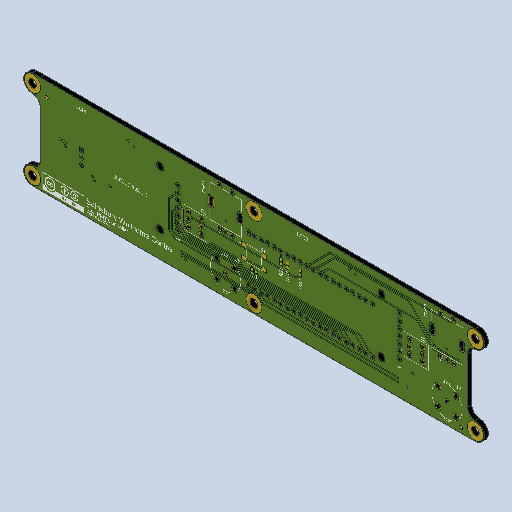
# Autodesk Inventor part: Dual PMT Controller_BOARD
Saved by Autodesk Inventor 2023 (Build 270158000, 158)
## iProperties
Created: 2023-07-11
Part Number: Dual PMT Controller_BOARD
Material: Generic
Document SubType Name: Modeling
Designer: Graeme
Density: 1 g/cm^3
Appearance: BoardColor
Author: Graeme
Autodesk Inventor part; units mm, degrees
ref_plane "YZ Plane" through (0, 0, 0) normal (1, 0, 0) x (0, 1, 0)
ref_plane "XZ Plane" through (0, 0, 0) normal (0, 1, 0) x (-1, 0, 0)
ref_plane "BoardFrontPlane" through (0, 0, 0) normal (0, 0, 1) x (1, 0, 0)
sketch "Sketch1" plane through (0, 0, 0) normal (0, 0, 1) x (1, 0, 0)
  line L0 (25, 25) -> (28, 25)
  line L1 (28, 25) -> (194, 25)
  line L2 (194, 25) -> (197, 25)
  arc A0 (197, 25) -> (197, 32) centre (197, 28.5) ccw
  arc A1 (194, 35) -> (197, 32) centre (197, 35) ccw
  line L3 (194, 35) -> (194, 53)
  arc A2 (197, 56) -> (194, 53) centre (197, 53) ccw
  arc A3 (197, 56) -> (197, 63) centre (197, 59.5) ccw
  line L4 (197, 63) -> (194, 63)
  line L5 (194, 63) -> (28, 63)
  line L6 (28, 63) -> (25, 63)
  arc A4 (25, 63) -> (25, 56) centre (25, 59.5) ccw
  arc A5 (28, 53) -> (25, 56) centre (25, 53) ccw
  line L7 (28, 53) -> (28, 35)
  arc A6 (25, 32) -> (28, 35) centre (25, 35) ccw
  arc A7 (25, 32) -> (25, 25) centre (25, 28.5) ccw
  constraints: 16 end point, 16 point on circle, 8 centre point
extrude "BoardOutline" add sketch "Sketch1" along normal blind 1.5954
sketch "Sketch4" plane through (0, 0, 1.5954) normal (0, 0, 1) x (1, 0, 0)
  line L0 (105.7, 53.45) -> (105.7, 55.55) construction
  line L1 (106.4, 53.45) -> (106.4, 55.55)
  line L2 (105, 55.55) -> (105, 53.45)
  arc A0 (105, 53.45) -> (106.4, 53.45) centre (105.7, 53.45) ccw
  arc A1 (106.4, 55.55) -> (105, 55.55) centre (105.7, 55.55) ccw
  point P0 (105.7, 54.5)
  constraints: 8 end point, 4 point on circle, 4 tangent, 2 centre point, 1 midpoint, 1 parallel
extrude "ENC1-4" cut sketch "Sketch4" against normal through all
sketch "Sketch5" plane through (0, 0, 1.5954) normal (0, 0, 1) x (1, 0, 0)
  line L0 (94.3, 53.45) -> (94.3, 55.55) construction
  line L1 (95, 53.45) -> (95, 55.55)
  line L2 (93.6, 55.55) -> (93.6, 53.45)
  arc A0 (93.6, 53.45) -> (95, 53.45) centre (94.3, 53.45) ccw
  arc A1 (95, 55.55) -> (93.6, 55.55) centre (94.3, 55.55) ccw
  point P0 (94.3, 54.5)
  constraints: 8 end point, 4 point on circle, 4 tangent, 2 centre point, 1 midpoint, 1 parallel
extrude "ENC1-3" cut sketch "Sketch5" against normal through all
sketch "Sketch6" plane through (0, 0, 1.5954) normal (0, 0, 1) x (1, 0, 0)
  point P0 (102.5, 47)
hole "ENC1-B" at (102.5, 47, 1.5954) direction (0, 0, -1) diameter 1 end through all
sketch "Sketch7" plane through (0, 0, 1.5954) normal (0, 0, 1) x (1, 0, 0)
  point P0 (100, 47)
hole "ENC1-C" at (100, 47, 1.5954) direction (0, 0, -1) diameter 1 end through all
sketch "Sketch8" plane through (0, 0, 1.5954) normal (0, 0, 1) x (1, 0, 0)
  point P0 (97.5, 47)
hole "ENC1-A" at (97.5, 47, 1.5954) direction (0, 0, -1) diameter 1 end through all
sketch "Sketch9" plane through (0, 0, 1.5954) normal (0, 0, 1) x (1, 0, 0)
  point P0 (102.5, 61.5)
hole "ENC1-2" at (102.5, 61.5, 1.5954) direction (0, 0, -1) diameter 1 end through all
sketch "Sketch10" plane through (0, 0, 1.5954) normal (0, 0, 1) x (1, 0, 0)
  point P0 (97.5, 61.5)
hole "ENC1-1" at (97.5, 61.5, 1.5954) direction (0, 0, -1) diameter 1 end through all
sketch "Sketch11" plane through (0, 0, 1.5954) normal (0, 0, 1) x (1, 0, 0)
  line L0 (191.7, 53.45) -> (191.7, 55.55) construction
  line L1 (192.4, 53.45) -> (192.4, 55.55)
  line L2 (191, 55.55) -> (191, 53.45)
  arc A0 (191, 53.45) -> (192.4, 53.45) centre (191.7, 53.45) ccw
  arc A1 (192.4, 55.55) -> (191, 55.55) centre (191.7, 55.55) ccw
  point P0 (191.7, 54.5)
  constraints: 8 end point, 4 point on circle, 4 tangent, 2 centre point, 1 midpoint, 1 parallel
extrude "ENC2-4" cut sketch "Sketch11" against normal through all
sketch "Sketch12" plane through (0, 0, 1.5954) normal (0, 0, 1) x (1, 0, 0)
  line L0 (180.3, 53.45) -> (180.3, 55.55) construction
  line L1 (181, 53.45) -> (181, 55.55)
  line L2 (179.6, 55.55) -> (179.6, 53.45)
  arc A0 (179.6, 53.45) -> (181, 53.45) centre (180.3, 53.45) ccw
  arc A1 (181, 55.55) -> (179.6, 55.55) centre (180.3, 55.55) ccw
  point P0 (180.3, 54.5)
  constraints: 8 end point, 4 point on circle, 4 tangent, 2 centre point, 1 midpoint, 1 parallel
extrude "ENC2-3" cut sketch "Sketch12" against normal through all
sketch "Sketch13" plane through (0, 0, 1.5954) normal (0, 0, 1) x (1, 0, 0)
  point P0 (188.5, 47)
hole "ENC2-B" at (188.5, 47, 1.5954) direction (0, 0, -1) diameter 1 end through all
sketch "Sketch14" plane through (0, 0, 1.5954) normal (0, 0, 1) x (1, 0, 0)
  point P0 (186, 47)
hole "ENC2-C" at (186, 47, 1.5954) direction (0, 0, -1) diameter 1 end through all
sketch "Sketch15" plane through (0, 0, 1.5954) normal (0, 0, 1) x (1, 0, 0)
  point P0 (183.5, 47)
hole "ENC2-A" at (183.5, 47, 1.5954) direction (0, 0, -1) diameter 1 end through all
sketch "Sketch16" plane through (0, 0, 1.5954) normal (0, 0, 1) x (1, 0, 0)
  point P0 (188.5, 61.5)
hole "ENC2-2" at (188.5, 61.5, 1.5954) direction (0, 0, -1) diameter 1 end through all
sketch "Sketch17" plane through (0, 0, 1.5954) normal (0, 0, 1) x (1, 0, 0)
  point P0 (183.5, 61.5)
hole "ENC2-1" at (183.5, 61.5, 1.5954) direction (0, 0, -1) diameter 1 end through all
sketch "Sketch18" plane through (0, 0, 1.5954) normal (0, 0, 1) x (1, 0, 0)
  point P0 (100, 33)
hole "J9-1" at (100, 33, 1.5954) direction (0, 0, -1) diameter 0.9906 end through all
sketch "Sketch19" plane through (0, 0, 1.5954) normal (0, 0, 1) x (1, 0, 0)
  point P0 (96.5583, 36.4417)
hole "J9-2" at (96.5583, 36.4417, 1.5954) direction (0, 0, -1) diameter 1.4986 end through all
sketch "Sketch20" plane through (0, 0, 1.5954) normal (0, 0, 1) x (1, 0, 0)
  point P0 (103.4417, 36.4417)
hole "J9-3" at (103.4417, 36.4417, 1.5954) direction (0, 0, -1) diameter 1.4986 end through all
sketch "Sketch21" plane through (0, 0, 1.5954) normal (0, 0, 1) x (1, 0, 0)
  point P0 (96.5583, 29.5583)
hole "J9-4" at (96.5583, 29.5583, 1.5954) direction (0, 0, -1) diameter 1.4986 end through all
sketch "Sketch22" plane through (0, 0, 1.5954) normal (0, 0, 1) x (1, 0, 0)
  point P0 (103.4417, 29.5583)
hole "J9-5" at (103.4417, 29.5583, 1.5954) direction (0, 0, -1) diameter 1.4986 end through all
sketch "Sketch23" plane through (0, 0, 1.5954) normal (0, 0, 1) x (1, 0, 0)
  point P0 (186, 33)
hole "J7-1" at (186, 33, 1.5954) direction (0, 0, -1) diameter 0.9906 end through all
sketch "Sketch24" plane through (0, 0, 1.5954) normal (0, 0, 1) x (1, 0, 0)
  point P0 (182.5583, 36.4417)
hole "J7-2" at (182.5583, 36.4417, 1.5954) direction (0, 0, -1) diameter 1.4986 end through all
sketch "Sketch25" plane through (0, 0, 1.5954) normal (0, 0, 1) x (1, 0, 0)
  point P0 (189.4417, 36.4417)
hole "J7-3" at (189.4417, 36.4417, 1.5954) direction (0, 0, -1) diameter 1.4986 end through all
sketch "Sketch26" plane through (0, 0, 1.5954) normal (0, 0, 1) x (1, 0, 0)
  point P0 (182.5583, 29.5583)
hole "J7-4" at (182.5583, 29.5583, 1.5954) direction (0, 0, -1) diameter 1.4986 end through all
sketch "Sketch27" plane through (0, 0, 1.5954) normal (0, 0, 1) x (1, 0, 0)
  point P0 (189.4417, 29.5583)
hole "J7-5" at (189.4417, 29.5583, 1.5954) direction (0, 0, -1) diameter 1.4986 end through all
sketch "Sketch28" plane through (0, 0, 1.5954) normal (0, 0, 1) x (1, 0, 0)
  point P0 (85.5, 41.46)
hole "S3-1" at (85.5, 41.46, 1.5954) direction (0, 0, -1) diameter 1.09 end through all
sketch "Sketch29" plane through (0, 0, 1.5954) normal (0, 0, 1) x (1, 0, 0)
  point P0 (85.5, 44)
hole "S3-2" at (85.5, 44, 1.5954) direction (0, 0, -1) diameter 1.09 end through all
sketch "Sketch30" plane through (0, 0, 1.5954) normal (0, 0, 1) x (1, 0, 0)
  point P0 (85.5, 46.54)
hole "S3-3" at (85.5, 46.54, 1.5954) direction (0, 0, -1) diameter 1.09 end through all
sketch "Sketch31" plane through (0, 0, 1.5954) normal (0, 0, 1) x (1, 0, 0)
  point P0 (90.58, 41.46)
hole "S3-4" at (90.58, 41.46, 1.5954) direction (0, 0, -1) diameter 1.09 end through all
sketch "Sketch32" plane through (0, 0, 1.5954) normal (0, 0, 1) x (1, 0, 0)
  point P0 (90.58, 44)
hole "S3-5" at (90.58, 44, 1.5954) direction (0, 0, -1) diameter 1.09 end through all
sketch "Sketch33" plane through (0, 0, 1.5954) normal (0, 0, 1) x (1, 0, 0)
  point P0 (90.58, 46.54)
hole "S3-6" at (90.58, 46.54, 1.5954) direction (0, 0, -1) diameter 1.09 end through all
sketch "Sketch34" plane through (0, 0, 1.5954) normal (0, 0, 1) x (1, 0, 0)
  point P0 (171.5, 41.46)
hole "S2-1" at (171.5, 41.46, 1.5954) direction (0, 0, -1) diameter 1.09 end through all
sketch "Sketch35" plane through (0, 0, 1.5954) normal (0, 0, 1) x (1, 0, 0)
  point P0 (171.5, 44)
hole "S2-2" at (171.5, 44, 1.5954) direction (0, 0, -1) diameter 1.09 end through all
sketch "Sketch36" plane through (0, 0, 1.5954) normal (0, 0, 1) x (1, 0, 0)
  point P0 (171.5, 46.54)
hole "S2-3" at (171.5, 46.54, 1.5954) direction (0, 0, -1) diameter 1.09 end through all
sketch "Sketch37" plane through (0, 0, 1.5954) normal (0, 0, 1) x (1, 0, 0)
  point P0 (176.58, 41.46)
hole "S2-4" at (176.58, 41.46, 1.5954) direction (0, 0, -1) diameter 1.09 end through all
sketch "Sketch38" plane through (0, 0, 1.5954) normal (0, 0, 1) x (1, 0, 0)
  point P0 (176.58, 44)
hole "S2-5" at (176.58, 44, 1.5954) direction (0, 0, -1) diameter 1.09 end through all
sketch "Sketch39" plane through (0, 0, 1.5954) normal (0, 0, 1) x (1, 0, 0)
  point P0 (176.58, 46.54)
hole "S2-6" at (176.58, 46.54, 1.5954) direction (0, 0, -1) diameter 1.09 end through all
sketch "Sketch40" plane through (0, 0, 1.5954) normal (0, 0, 1) x (1, 0, 0)
  point P0 (81.48, 53.38)
hole "LCD1-7" at (81.48, 53.38, 1.5954) direction (0, 0, -1) diameter 1 end through all
sketch "Sketch41" plane through (0, 0, 1.5954) normal (0, 0, 1) x (1, 0, 0)
  point P0 (81.48, 50.84)
hole "LCD1-6" at (81.48, 50.84, 1.5954) direction (0, 0, -1) diameter 1 end through all
sketch "Sketch42" plane through (0, 0, 1.5954) normal (0, 0, 1) x (1, 0, 0)
  point P0 (81.48, 48.3)
hole "LCD1-5" at (81.48, 48.3, 1.5954) direction (0, 0, -1) diameter 1 end through all
sketch "Sketch43" plane through (0, 0, 1.5954) normal (0, 0, 1) x (1, 0, 0)
  point P0 (81.48, 45.76)
hole "LCD1-4" at (81.48, 45.76, 1.5954) direction (0, 0, -1) diameter 1 end through all
sketch "Sketch44" plane through (0, 0, 1.5954) normal (0, 0, 1) x (1, 0, 0)
  point P0 (81.48, 43.22)
hole "LCD1-3" at (81.48, 43.22, 1.5954) direction (0, 0, -1) diameter 1 end through all
sketch "Sketch45" plane through (0, 0, 1.5954) normal (0, 0, 1) x (1, 0, 0)
  point P0 (81.48, 40.68)
hole "LCD1-2" at (81.48, 40.68, 1.5954) direction (0, 0, -1) diameter 1 end through all
sketch "Sketch46" plane through (0, 0, 1.5954) normal (0, 0, 1) x (1, 0, 0)
  point P0 (81.48, 38.14)
hole "LCD1-1" at (81.48, 38.14, 1.5954) direction (0, 0, -1) diameter 1 end through all
sketch "Sketch47" plane through (0, 0, 1.5954) normal (0, 0, 1) x (1, 0, 0)
  point P0 (74.58, 56.36)
hole "LCD1-MH1" at (74.58, 56.36, 1.5954) direction (0, 0, -1) diameter 2.5 end through all
sketch "Sketch48" plane through (0, 0, 1.5954) normal (0, 0, 1) x (1, 0, 0)
  point P0 (74.58, 35.16)
hole "LCD1-MH2" at (74.58, 35.16, 1.5954) direction (0, 0, -1) diameter 2.5 end through all
sketch "Sketch49" plane through (0, 0, 1.5954) normal (0, 0, 1) x (1, 0, 0)
  point P0 (167.48, 53.38)
hole "LCD2-7" at (167.48, 53.38, 1.5954) direction (0, 0, -1) diameter 1 end through all
sketch "Sketch50" plane through (0, 0, 1.5954) normal (0, 0, 1) x (1, 0, 0)
  point P0 (167.48, 50.84)
hole "LCD2-6" at (167.48, 50.84, 1.5954) direction (0, 0, -1) diameter 1 end through all
sketch "Sketch51" plane through (0, 0, 1.5954) normal (0, 0, 1) x (1, 0, 0)
  point P0 (167.48, 48.3)
hole "LCD2-5" at (167.48, 48.3, 1.5954) direction (0, 0, -1) diameter 1 end through all
sketch "Sketch52" plane through (0, 0, 1.5954) normal (0, 0, 1) x (1, 0, 0)
  point P0 (167.48, 45.76)
hole "LCD2-4" at (167.48, 45.76, 1.5954) direction (0, 0, -1) diameter 1 end through all
sketch "Sketch53" plane through (0, 0, 1.5954) normal (0, 0, 1) x (1, 0, 0)
  point P0 (167.48, 43.22)
hole "LCD2-3" at (167.48, 43.22, 1.5954) direction (0, 0, -1) diameter 1 end through all
sketch "Sketch54" plane through (0, 0, 1.5954) normal (0, 0, 1) x (1, 0, 0)
  point P0 (167.48, 40.68)
hole "LCD2-2" at (167.48, 40.68, 1.5954) direction (0, 0, -1) diameter 1 end through all
sketch "Sketch55" plane through (0, 0, 1.5954) normal (0, 0, 1) x (1, 0, 0)
  point P0 (167.48, 38.14)
hole "LCD2-1" at (167.48, 38.14, 1.5954) direction (0, 0, -1) diameter 1 end through all
sketch "Sketch56" plane through (0, 0, 1.5954) normal (0, 0, 1) x (1, 0, 0)
  point P0 (160.58, 56.36)
hole "LCD2-MH1" at (160.58, 56.36, 1.5954) direction (0, 0, -1) diameter 2.5 end through all
sketch "Sketch57" plane through (0, 0, 1.5954) normal (0, 0, 1) x (1, 0, 0)
  point P0 (160.58, 35.16)
hole "LCD2-MH2" at (160.58, 35.16, 1.5954) direction (0, 0, -1) diameter 2.5 end through all
sketch "Sketch98" plane through (0, 0, 1.5954) normal (0, 0, 1) x (1, 0, 0)
  point P0 (44, 46.54)
hole "PS1-1" at (44, 46.54, 1.5954) direction (0, 0, -1) diameter 0.85 end through all
sketch "Sketch99" plane through (0, 0, 1.5954) normal (0, 0, 1) x (1, 0, 0)
  point P0 (44, 44)
hole "PS1-2" at (44, 44, 1.5954) direction (0, 0, -1) diameter 0.85 end through all
sketch "Sketch100" plane through (0, 0, 1.5954) normal (0, 0, 1) x (1, 0, 0)
  point P0 (44, 41.46)
hole "PS1-3" at (44, 41.46, 1.5954) direction (0, 0, -1) diameter 0.85 end through all
sketch "Sketch101" plane through (0, 0, 1.5954) normal (0, 0, 1) x (1, 0, 0)
  point P0 (25, 59.5)
hole "Free-MH1_LWOVBYDG" at (25, 59.5, 1.5954) direction (0, 0, -1) diameter 3.1 end through all
sketch "Sketch102" plane through (0, 0, 1.5954) normal (0, 0, 1) x (1, 0, 0)
  point P0 (25, 28.5)
hole "Free-MH1_XUCMYAUQ" at (25, 28.5, 1.5954) direction (0, 0, -1) diameter 3.1 end through all
sketch "Sketch103" plane through (0, 0, 1.5954) normal (0, 0, 1) x (1, 0, 0)
  point P0 (111, 28.5)
hole "Free-MH1_AHOANEHU" at (111, 28.5, 1.5954) direction (0, 0, -1) diameter 3.1 end through all
sketch "Sketch104" plane through (0, 0, 1.5954) normal (0, 0, 1) x (1, 0, 0)
  point P0 (111, 59.5)
hole "Free-MH1_SKXHPFAL" at (111, 59.5, 1.5954) direction (0, 0, -1) diameter 3.1 end through all
sketch "Sketch105" plane through (0, 0, 1.5954) normal (0, 0, 1) x (1, 0, 0)
  point P0 (197, 28.5)
hole "Free-MH1_TQVXVKIN" at (197, 28.5, 1.5954) direction (0, 0, -1) diameter 3.1 end through all
sketch "Sketch106" plane through (0, 0, 1.5954) normal (0, 0, 1) x (1, 0, 0)
  point P0 (197, 59.5)
hole "Free-MH1_OJOGQPHQ" at (197, 59.5, 1.5954) direction (0, 0, -1) diameter 3.1 end through all
sketch "img_Top" plane through (0, 0, 1.5954) normal (0, 0, 1) x (1, 0, 0)
  line L0 (21.5, 63) -> (200.5015, 63) construction
  line L1 (200.5015, 63) -> (200.5015, 25) construction
  line L2 (200.5015, 25) -> (21.5, 25) construction
  line L3 (21.5, 25) -> (21.5, 63) construction
  constraints: 2 other
decal "Decal_Top"
sketch "img_Bottom" plane through (0, 0, -1.5954) normal (0, 0, -1) x (1, 0, 0)
  line L0 (21.5, -25) -> (200.5015, -25) construction
  line L1 (200.5015, -25) -> (200.5015, -63) construction
  line L2 (200.5015, -63) -> (21.5, -63) construction
  line L3 (21.5, -63) -> (21.5, -25) construction
  constraints: 2 other
decal "Decal_Bottom"
sketch "Sketch109" plane through (0, 0, 1.5954) normal (0, 0, 1) x (1, 0, 0)
  point P0 (157.01, 51.28)
hole "J1-20" at (157.01, 51.28, 1.5954) direction (0, 0, -1) diameter 1.04 end through all
sketch "Sketch110" plane through (0, 0, 1.5954) normal (0, 0, 1) x (1, 0, 0)
  point P0 (154.47, 51.28)
hole "J1-19" at (154.47, 51.28, 1.5954) direction (0, 0, -1) diameter 1.04 end through all
sketch "Sketch111" plane through (0, 0, 1.5954) normal (0, 0, 1) x (1, 0, 0)
  point P0 (151.93, 51.28)
hole "J1-18" at (151.93, 51.28, 1.5954) direction (0, 0, -1) diameter 1.04 end through all
sketch "Sketch112" plane through (0, 0, 1.5954) normal (0, 0, 1) x (1, 0, 0)
  point P0 (149.39, 51.28)
hole "J1-17" at (149.39, 51.28, 1.5954) direction (0, 0, -1) diameter 1.04 end through all
sketch "Sketch113" plane through (0, 0, 1.5954) normal (0, 0, 1) x (1, 0, 0)
  point P0 (146.85, 51.28)
hole "J1-16" at (146.85, 51.28, 1.5954) direction (0, 0, -1) diameter 1.04 end through all
sketch "Sketch114" plane through (0, 0, 1.5954) normal (0, 0, 1) x (1, 0, 0)
  point P0 (144.31, 51.28)
hole "J1-15" at (144.31, 51.28, 1.5954) direction (0, 0, -1) diameter 1.04 end through all
sketch "Sketch115" plane through (0, 0, 1.5954) normal (0, 0, 1) x (1, 0, 0)
  point P0 (141.77, 51.28)
hole "J1-14" at (141.77, 51.28, 1.5954) direction (0, 0, -1) diameter 1.04 end through all
sketch "Sketch116" plane through (0, 0, 1.5954) normal (0, 0, 1) x (1, 0, 0)
  point P0 (139.23, 51.28)
hole "J1-13" at (139.23, 51.28, 1.5954) direction (0, 0, -1) diameter 1.04 end through all
sketch "Sketch117" plane through (0, 0, 1.5954) normal (0, 0, 1) x (1, 0, 0)
  point P0 (136.69, 51.28)
hole "J1-12" at (136.69, 51.28, 1.5954) direction (0, 0, -1) diameter 1.04 end through all
sketch "Sketch118" plane through (0, 0, 1.5954) normal (0, 0, 1) x (1, 0, 0)
  point P0 (134.15, 51.28)
hole "J1-11" at (134.15, 51.28, 1.5954) direction (0, 0, -1) diameter 1.04 end through all
sketch "Sketch119" plane through (0, 0, 1.5954) normal (0, 0, 1) x (1, 0, 0)
  point P0 (131.61, 51.28)
hole "J1-10" at (131.61, 51.28, 1.5954) direction (0, 0, -1) diameter 1.04 end through all
sketch "Sketch120" plane through (0, 0, 1.5954) normal (0, 0, 1) x (1, 0, 0)
  point P0 (129.07, 51.28)
hole "J1-9" at (129.07, 51.28, 1.5954) direction (0, 0, -1) diameter 1.04 end through all
sketch "Sketch121" plane through (0, 0, 1.5954) normal (0, 0, 1) x (1, 0, 0)
  point P0 (126.53, 51.28)
hole "J1-8" at (126.53, 51.28, 1.5954) direction (0, 0, -1) diameter 1.04 end through all
sketch "Sketch122" plane through (0, 0, 1.5954) normal (0, 0, 1) x (1, 0, 0)
  point P0 (123.99, 51.28)
hole "J1-7" at (123.99, 51.28, 1.5954) direction (0, 0, -1) diameter 1.04 end through all
sketch "Sketch123" plane through (0, 0, 1.5954) normal (0, 0, 1) x (1, 0, 0)
  point P0 (121.45, 51.28)
hole "J1-6" at (121.45, 51.28, 1.5954) direction (0, 0, -1) diameter 1.04 end through all
sketch "Sketch124" plane through (0, 0, 1.5954) normal (0, 0, 1) x (1, 0, 0)
  point P0 (118.91, 51.28)
hole "J1-5" at (118.91, 51.28, 1.5954) direction (0, 0, -1) diameter 1.04 end through all
sketch "Sketch125" plane through (0, 0, 1.5954) normal (0, 0, 1) x (1, 0, 0)
  point P0 (116.37, 51.28)
hole "J1-4" at (116.37, 51.28, 1.5954) direction (0, 0, -1) diameter 1.04 end through all
sketch "Sketch126" plane through (0, 0, 1.5954) normal (0, 0, 1) x (1, 0, 0)
  point P0 (113.83, 51.28)
hole "J1-3" at (113.83, 51.28, 1.5954) direction (0, 0, -1) diameter 1.04 end through all
sketch "Sketch127" plane through (0, 0, 1.5954) normal (0, 0, 1) x (1, 0, 0)
  point P0 (111.29, 51.28)
hole "J1-2" at (111.29, 51.28, 1.5954) direction (0, 0, -1) diameter 1.04 end through all
sketch "Sketch128" plane through (0, 0, 1.5954) normal (0, 0, 1) x (1, 0, 0)
  point P0 (108.75, 51.28)
hole "J1-1" at (108.75, 51.28, 1.5954) direction (0, 0, -1) diameter 1.04 end through all
sketch "Sketch129" plane through (0, 0, 1.5954) normal (0, 0, 1) x (1, 0, 0)
  point P0 (108.75, 33.5)
hole "J2-40" at (108.75, 33.5, 1.5954) direction (0, 0, -1) diameter 1.04 end through all
sketch "Sketch130" plane through (0, 0, 1.5954) normal (0, 0, 1) x (1, 0, 0)
  point P0 (111.29, 33.5)
hole "J2-39" at (111.29, 33.5, 1.5954) direction (0, 0, -1) diameter 1.04 end through all
sketch "Sketch131" plane through (0, 0, 1.5954) normal (0, 0, 1) x (1, 0, 0)
  point P0 (113.83, 33.5)
hole "J2-38" at (113.83, 33.5, 1.5954) direction (0, 0, -1) diameter 1.04 end through all
sketch "Sketch132" plane through (0, 0, 1.5954) normal (0, 0, 1) x (1, 0, 0)
  point P0 (116.37, 33.5)
hole "J2-37" at (116.37, 33.5, 1.5954) direction (0, 0, -1) diameter 1.04 end through all
sketch "Sketch133" plane through (0, 0, 1.5954) normal (0, 0, 1) x (1, 0, 0)
  point P0 (118.91, 33.5)
hole "J2-36" at (118.91, 33.5, 1.5954) direction (0, 0, -1) diameter 1.04 end through all
sketch "Sketch134" plane through (0, 0, 1.5954) normal (0, 0, 1) x (1, 0, 0)
  point P0 (121.45, 33.5)
hole "J2-35" at (121.45, 33.5, 1.5954) direction (0, 0, -1) diameter 1.04 end through all
sketch "Sketch135" plane through (0, 0, 1.5954) normal (0, 0, 1) x (1, 0, 0)
  point P0 (123.99, 33.5)
hole "J2-34" at (123.99, 33.5, 1.5954) direction (0, 0, -1) diameter 1.04 end through all
sketch "Sketch136" plane through (0, 0, 1.5954) normal (0, 0, 1) x (1, 0, 0)
  point P0 (126.53, 33.5)
hole "J2-33" at (126.53, 33.5, 1.5954) direction (0, 0, -1) diameter 1.04 end through all
sketch "Sketch137" plane through (0, 0, 1.5954) normal (0, 0, 1) x (1, 0, 0)
  point P0 (129.07, 33.5)
hole "J2-32" at (129.07, 33.5, 1.5954) direction (0, 0, -1) diameter 1.04 end through all
sketch "Sketch138" plane through (0, 0, 1.5954) normal (0, 0, 1) x (1, 0, 0)
  point P0 (131.61, 33.5)
hole "J2-31" at (131.61, 33.5, 1.5954) direction (0, 0, -1) diameter 1.04 end through all
sketch "Sketch139" plane through (0, 0, 1.5954) normal (0, 0, 1) x (1, 0, 0)
  point P0 (134.15, 33.5)
hole "J2-30" at (134.15, 33.5, 1.5954) direction (0, 0, -1) diameter 1.04 end through all
sketch "Sketch140" plane through (0, 0, 1.5954) normal (0, 0, 1) x (1, 0, 0)
  point P0 (136.69, 33.5)
hole "J2-29" at (136.69, 33.5, 1.5954) direction (0, 0, -1) diameter 1.04 end through all
sketch "Sketch141" plane through (0, 0, 1.5954) normal (0, 0, 1) x (1, 0, 0)
  point P0 (139.23, 33.5)
hole "J2-28" at (139.23, 33.5, 1.5954) direction (0, 0, -1) diameter 1.04 end through all
sketch "Sketch142" plane through (0, 0, 1.5954) normal (0, 0, 1) x (1, 0, 0)
  point P0 (141.77, 33.5)
hole "J2-27" at (141.77, 33.5, 1.5954) direction (0, 0, -1) diameter 1.04 end through all
sketch "Sketch143" plane through (0, 0, 1.5954) normal (0, 0, 1) x (1, 0, 0)
  point P0 (144.31, 33.5)
hole "J2-26" at (144.31, 33.5, 1.5954) direction (0, 0, -1) diameter 1.04 end through all
sketch "Sketch144" plane through (0, 0, 1.5954) normal (0, 0, 1) x (1, 0, 0)
  point P0 (146.85, 33.5)
hole "J2-25" at (146.85, 33.5, 1.5954) direction (0, 0, -1) diameter 1.04 end through all
sketch "Sketch145" plane through (0, 0, 1.5954) normal (0, 0, 1) x (1, 0, 0)
  point P0 (149.39, 33.5)
hole "J2-24" at (149.39, 33.5, 1.5954) direction (0, 0, -1) diameter 1.04 end through all
sketch "Sketch146" plane through (0, 0, 1.5954) normal (0, 0, 1) x (1, 0, 0)
  point P0 (151.93, 33.5)
hole "J2-23" at (151.93, 33.5, 1.5954) direction (0, 0, -1) diameter 1.04 end through all
sketch "Sketch147" plane through (0, 0, 1.5954) normal (0, 0, 1) x (1, 0, 0)
  point P0 (154.47, 33.5)
hole "J2-22" at (154.47, 33.5, 1.5954) direction (0, 0, -1) diameter 1.04 end through all
sketch "Sketch148" plane through (0, 0, 1.5954) normal (0, 0, 1) x (1, 0, 0)
  point P0 (157.01, 33.5)
hole "J2-21" at (157.01, 33.5, 1.5954) direction (0, 0, -1) diameter 1.04 end through all
body "Solid1"
